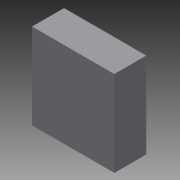
# Autodesk Inventor part: LED
Saved by Autodesk Inventor 2015 SP2 (Build 190223200, 223)
## iProperties
Created: 2024-01-08
Part Number: LED
Material: Generisch
Document SubType Name: Modeling
Designer: montag01
Density: 1 g/cm^3
Appearance: Vorgabe
Author: montag01
Autodesk Inventor part; units mm, degrees
ref_plane "YZ Plane" through (0, 0, 0) normal (1, 0, 0) x (0, 1, 0)
ref_plane "XZ Plane" through (0, 0, 0) normal (0, 1, 0) x (-1, 0, 0)
ref_plane "XY Plane" through (0, 0, 0) normal (0, 0, 1) x (1, 0, 0)
sketch "Skizze1" plane through (0, 0, 0) normal (0, 1, 0) x (-1, 0, 0)
  line L0 (0, 0) -> (0, -5.1)
  line L1 (0, -5.1) -> (4.9, -5.1)
  line L2 (4.9, -5.1) -> (4.9, 0)
  line L3 (4.9, 0) -> (0, 0)
  dimension "d0" = 5.1
  dimension "d1" = 4.9
  constraints: 8 end point, 3 perpendicular, 1 vertical
  measures "d0" distance of L0.start L0.end
  measures "d1" distance of L0.end L1.end
extrude "Extrusion1" add sketch "Skizze1" along normal blind 2
fillet "Rundung1" radius 0.15 4 edges at (-2.45, 2, 0) (0, 2, -2.55) (-2.45, 2, -5.1) (-4.9, 2, -2.55)
